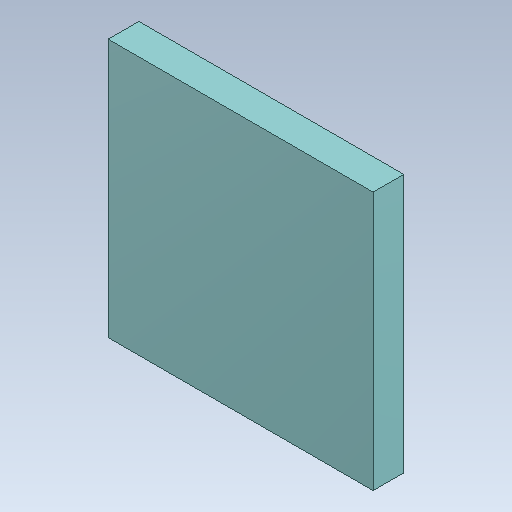
# Autodesk Inventor part: TCA9548APWR
Saved by Autodesk Inventor 2020 (Build 240168000, 168)
## iProperties
Created: 2019-08-29
Part Number: TCA9548APWR
Material: Generic
Document SubType Name: Modeling
Designer: psrob
Density: 1 g/cm^3
Appearance: SOP65P640X120-24N, TCA9548APWR
Author: psrob
Autodesk Inventor part; units mm, degrees
ref_plane "YZ Plane" through (0, 0, 0) normal (1, 0, 0) x (0, 1, 0)
ref_plane "XZ Plane" through (0, 0, 0) normal (0, 1, 0) x (-1, 0, 0)
ref_plane "XY Plane" through (0, 0, 0) normal (0, 0, 1) x (1, 0, 0)
sketch "SOP65P640X120-24N, TCA9548APWR_46" plane through (0, 0, 0) normal (0, 0, 1) x (1, 0, 0)
  line L0 (-4.725, 4.27) -> (3.905, 4.27)
  line L1 (3.905, 4.27) -> (3.905, -4.15)
  line L2 (3.905, -4.15) -> (-4.725, -4.15)
  line L3 (-4.725, -4.15) -> (-4.725, 4.27)
  constraints: 8 end point
extrude "Extrusion1" add sketch "SOP65P640X120-24N, TCA9548APWR_46" along normal blind 1
body "Solid1"
